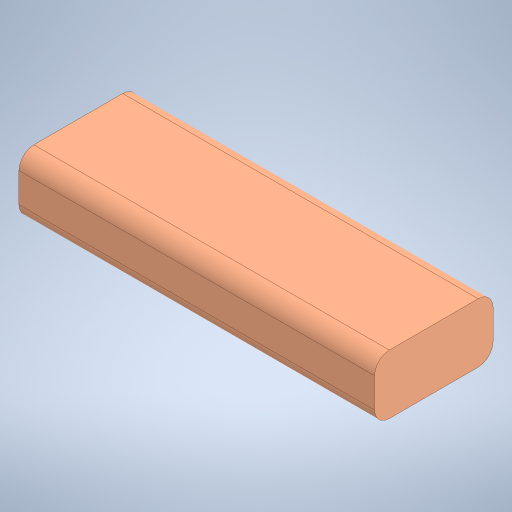
# Autodesk Inventor part: Wood-3
Saved by Autodesk Inventor 2024 (Build 280153000, 153)
## iProperties
Created: 2024-03-20
Part Number: Wood-3
Material: Generic
Document SubType Name: Modeling
Designer: Liz
Density: 1 g/cm^3
Appearance: Default
Author: Liz
Autodesk Inventor part; units mm, degrees
ref_plane "YZ Plane" through (0, 0, 0) normal (1, 0, 0) x (0, 1, 0)
ref_plane "XZ Plane" through (0, 0, 0) normal (0, 1, 0) x (-1, 0, 0)
ref_plane "XY Plane" through (0, 0, 0) normal (0, 0, 1) x (1, 0, 0)
sketch "Sketch1" plane through (0, 0, 0) normal (1, 0, 0) x (0, 1, 0)
  line L0 (-12.7, 50.8) -> (12.7, 50.8)
  line L1 (25.4, 38.1) -> (25.4, -38.1)
  line L2 (12.7, -50.8) -> (-12.7, -50.8)
  line L3 (-25.4, -38.1) -> (-25.4, 38.1)
  line L4 (-25.4, 50.8) -> (25.4, -50.8) construction
  line L5 (25.4, 50.8) -> (-25.4, -50.8) construction
  arc A0 (25.4, 38.1) -> (12.7, 50.8) centre (12.7, 38.1) ccw
  arc A1 (-12.7, 50.8) -> (-25.4, 38.1) centre (-12.7, 38.1) ccw
  arc A2 (-25.4, -38.1) -> (-12.7, -50.8) centre (-12.7, -38.1) ccw
  arc A3 (12.7, -50.8) -> (25.4, -38.1) centre (12.7, -38.1) ccw
  point P0 (0, 0)
  dimension "d0" = 101.6
  dimension "d1" = 50.8
  dimension "d2" = 12.7
  constraints: 12 end point, 8 point on circle, 8 point on line, 8 tangent, 4 centre point, 3 equal radius, 2 midpoint, 2 parallel, 1 horizontal, 1 perpendicular
  measures "d0" distance of L5.start L4.end
  measures "d1" distance of L4.start L5.start
  measures "d2" radius of A0
extrude "Extrusion1" add sketch "Sketch1" against normal blind 304.8
body "Solid1"
